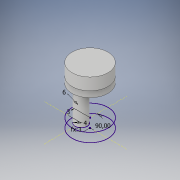
# Autodesk Inventor part: ExcentricShaft
Saved by Autodesk Inventor 2018.3 (Build 223284000, 284)
## iProperties
Created: 2018-07-20
Part Number: ExcentricShaft
Material: Generisch
Document SubType Name: Modeling
Designer: JochenAlt
Density: 1 g/cm^3
Appearance: Vorgabe
Author: JochenAlt
Autodesk Inventor part; units mm, degrees
ref_plane "YZ Plane" through (0, 0, 0) normal (1, 0, 0) x (0, 1, 0)
ref_plane "XZ Plane" through (0, 0, 0) normal (0, 1, 0) x (-1, 0, 0)
ref_plane "XY Plane" through (0, 0, 0) normal (0, 0, 1) x (1, 0, 0)
sketch "Skizze1" plane through (0, 0, 0) normal (0, 0, 1) x (1, 0, 0)
  line L0 (0, 15.4794) -> (0, -12.4794) construction
  line L1 (-12.4794, 0) -> (15.4794, 0) construction
  circle A0 centre (0, 0) radius 2
  arc A1 (-2.4686, -2.4686) -> (5.4686, 5.4686) centre (3, 0) ccw
  line L2 (0, 3) -> (0, 0) construction
  line L3 (0, 0) -> (3, 0) construction
  arc A2 (5.4686, 5.4686) -> (-2.4686, -2.4686) centre (0, 3) ccw
  arc A3 (-2.4686, -2.4686) -> (5.4686, 5.4686) centre (0, 3) ccw
  arc A4 (5.4686, 5.4686) -> (-2.4686, -2.4686) centre (3, 0) ccw
  line L4 (0, 0) -> (3, 0) construction
  dimension "d0" = 4
  dimension "d1" = 3
  dimension "d13" = 6
  dimension "d14" = 3
  dimension "d15" = 90
  constraints: 9 point on circle, 6 end point, 5 centre point, 3 equal radius, 2 collinear, 1 coincident, 1 concentric, 1 perpendicular, 1 point on line
  measures "d0" diameter of A0
  measures "d1" distance of point (0, 0) L2.start
  measures "d13" radius of A2
  measures "d14" distance of L2.end L4.end
  measures "d15" angle of L4 L0
extrude "Extrusion1" add sketch "Skizze1" along normal blind 10 contours A0
extrude "Extrusion2" add sketch "Skizze1" along normal blind 4 from surface at 10 contours A0 | A4 A3 | A2 A4
extrude "Extrusion3" add sketch "Skizze1" along normal blind 1 from surface at 14 contours A0 | A4 A3
extrude "Extrusion4" add sketch "Skizze1" along normal blind 4 from surface at 15 contours A0 | A3 A1 | A4 A3
equation "\"d14\" = d1"
